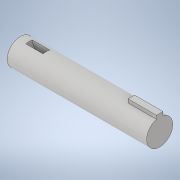
# Autodesk Inventor part: MotorShaft
Saved by Autodesk Inventor 2021 (Build 250183000, 183)
## iProperties
Created: 2020-09-20
Part Number: MotorShaft
Material: Generic
Document SubType Name: Modeling
Designer: PhotonUser
Density: 1 g/cm^3
Appearance: Default
Author: PhotonUser
Autodesk Inventor part; units mm, degrees
ref_plane "YZ Plane" through (0, 0, 0) normal (1, 0, 0) x (0, 1, 0)
ref_plane "XZ Plane" through (0, 0, 0) normal (0, 1, 0) x (-1, 0, 0)
ref_plane "XY Plane" through (0, 0, 0) normal (0, 0, 1) x (1, 0, 0)
sketch "Sketch1" plane through (0, 0, 0) normal (1, 0, 0) x (0, 1, 0)
  circle A0 centre (0, 0) radius 9.525
  dimension "d0" = 19.05
  constraints: 1 centre point, 1 coincident
  measures "d0" diameter of A0
extrude "Extrusion1" add sketch "Sketch1" along normal blind 101.6
sketch "Sketch2" plane through (101.6, 0, 0) normal (1, 0, 0) x (0, 0, -1)
  circle A0 centre (0, 0) radius 9.525 projected
  line L0 (-2.3876, 9.2209) -> (-2.3876, 11.7609)
  line L1 (-2.3876, 11.7609) -> (2.3876, 11.7609)
  line L2 (2.3876, 11.7609) -> (2.3876, 9.2209)
  line L3 (0, 0) -> (0, 17.2651)
  point P0 (0, 11.7609)
  dimension "d3" = 2.54
  dimension "d4" = 4.7752
  constraints: 8 end point, 2 perpendicular, 2 point on circle, 2 vertical, 1 midpoint, 1 point on line
  measures "d3" distance of L0.start L0.end
  measures "d4" distance between parallel lines of L2 L0
extrude "Extrusion2" add sketch "Sketch2" against normal blind 20.6502 contours A0 L3 L1 L2 | L0 L1 L3 A0
sketch "Sketch3" plane through (0, 0, 0) normal (0, 0, 1) x (1, 0, 0)
  line L0 (0, 9.525) -> (80.9498, 9.525) projected
  arc A0 (6.35, 9.525) -> (19.05, 9.525) centre (12.7, 9.525) ccw
  line L1 (6.35, 9.525) -> (19.05, 9.525)
  point P0 (0, 0)
  dimension "d7" = 12.7
  dimension "d8" = 12.7
  constraints: 3 point on line, 2 end point, 2 point on circle, 1 centre point
  measures "d7" distance of L0.start A0.centre
  measures "d8" diameter of A0
extrude "Extrusion3" cut sketch "Sketch3" against normal mid plane 4.7752
body "Solid1"
